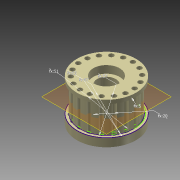
# Autodesk Inventor part: NagyKerek
Saved by Autodesk Inventor 2015 (Build 190159000, 159)
## iProperties
Created: 2014-04-13
Part Number: NagyKerek
Material: Nylon, molybdenum disulphide
Document SubType Name: Modeling
Designer: laca
Density: 1.13 g/cm^3
Appearance: Nylon 6
Mass: 91.8836 g
Surface Area: 251.529 cm^2
Volume: 81.3129 cm^3
Author: laca
Autodesk Inventor part; units mm, degrees
ref_plane "YZ Plane" through (0, 0, 0) normal (1, 0, 0) x (0, 1, 0)
ref_plane "XZ Plane" through (0, 0, 0) normal (0, 1, 0) x (-1, 0, 0)
ref_plane "XY Plane" through (0, 0, 0) normal (0, 0, 1) x (1, 0, 0)
sketch "Sketch1" plane through (0, 0, 0) normal (0, 0, 1) x (1, 0, 0)
  circle A0 centre (0.0338, 1.5) radius 28.5
  arc A1 (-1.1621, 26.972) -> (1.1984, 26.9734) centre (0.0338, 1.5) ccw
  line L0 (-1.1621, 26.972) -> (0.0338, 1.5)
  line L1 (0.0338, 1.5) -> (1.1984, 26.9734)
  arc A2 (1.3007, 29.9718) -> (-1.3028, 29.9687) centre (0.0338, 1.5) ccw
  circle A3 centre (1.3379, 26.9666) radius 2.5
  point P0 (1.3508, 29.9696)
  dimension "d53" = 5
  dimension "d22" = 57
  dimension "d23" = 51
  constraints: 8 point on circle, 4 end point, 3 centre point, 3 coincident, 3 other
  measures "d22" diameter of A0
  measures "d23" diameter of A1
sketch "Sketch2" plane through (0, 0, 0) normal (0, 0, 1) x (1, 0, 0)
  circle A0 centre (0, 0) radius 28.5
  circle A1 centre (0, 0) radius 10
  circle A2 centre (0, 0) radius 31.5
  dimension "d10" = 57
  dimension "d32" = 63
  dimension "d37" = 20
  constraints: 3 centre point, 3 coincident
  measures "d10" diameter of A0
  measures "d32" diameter of A2
  measures "d37" diameter of A1
extrude "Extrusion5" add sketch "Sketch2" along normal blind 31 contours A0
extrude "Extrusion9" add sketch "Sketch2" against normal blind 9 contours A0 | A2
sketch "Sketch3" plane through (0, 0, 31) normal (0, 0, 1) x (1, 0, 0)
  circle A0 centre (0, 0) radius 31.5
  circle A1 centre (0, 0) radius 10
  dimension "d38" = 63
  dimension "d40" = 20
  constraints: 2 centre point, 1 coincident
  measures "d38" diameter of A0
  measures "d40" diameter of A1
extrude "Extrusion11" add sketch "Sketch3" along normal blind 4
extrude "Extrusion15" cut sketch "Sketch1" along normal through all both and the other way through all contours A3 A1 L1 | A3 L1 A1
pattern_circular "Circular Pattern4" count 18 over 360 about axis through (0, 0, 0) along (0, 0, 1) of "Extrusion15"
sketch "Sketch7" plane through (0, 0, -9) normal (0, 0, -1) x (-1, 0, 0)
  circle A0 centre (0, 0) radius 10 projected
  circle A1 centre (0, 0) radius 31.5 projected
  circle A2 centre (0, 0) radius 14
  dimension "d62" = 28
  constraints: 1 centre point, 1 coincident
  measures "d62" diameter of A2
extrude "Extrusion17" cut sketch "Sketch7" against normal blind 27 contours A2
sketch "Sketch8" plane through (0, 0, 35) normal (0, 0, 1) x (1, 0, 0)
  circle A0 centre (0, 0) radius 14
  dimension "d65" = 28
  constraints: 1 centre point, 1 coincident
  measures "d65" diameter of A0
extrude "Extrusion18" cut sketch "Sketch8" against normal blind 8
ref_plane "Work Plane2" through (0, 0, 15.5) normal (0, 0, 1) x (1, 0, 0)
equation "\"d53\" = 2 * SzíjFogakSugaraA"
equation "\"d22\" = 0.5 * NagyKerekAtmero"
equation "\"d23\" = 0.5 * NagyKerekAtmero - 2 * SzíjSugarKözépontEltolásaAzAlaptolA"
equation "\"d10\" = 0.5 * NagyKerekAtmero"
equation "\"d32\" = 0.5 * NagyKerekAtmero + 2 * NagyKerekPeremMagasaga"
equation "\"d37\" = NgyKerekFurat"
equation "\"d15\" = SzíjSzélességB"
equation "\"d38\" = 0.5 * NagyKerekAtmero + 2 * NagyKerekPeremMagasaga"
equation "\"d40\" = NgyKerekFurat"
equation "\"d54\" = NagyKerekPeremSzélesege"
equation "\"d63\" = NagyKerekPeremSzélesege + 0.5 * SzíjSzélességB + 0.5 * KisKerekCSapagySzeleseg"
equation "\"SzíjSzélességA\" = 31"
equation "\"SzíjAlapVastagságA\" = 3"
equation "\"SzíjFogakSugaraA\" = 2.5"
equation "\"SzíjSugarKözépontEltolásaAzAlaptolA\" = 3"
equation "\"NagyKerekAtmero\" = 114"
equation "\"SzíjSzélességB\" = 31"
equation "\"SzíjFogakSugaraB\" = 2.5"
equation "\"SzíjSugarKözépontEltolásaAzAlaptolB\" = 3"
equation "\"SzíjAlapVastagságB\" = 3"
equation "\"NagyKerekPeremSzélesege\" = 4"
equation "\"NagyKerekPeremMagasaga\" = 3"
equation "\"NgyKerekFurat\" = 20"
equation "\"NagyKerekTengelyVastagsag\" = 14"
equation "\"NagyKerékCsapágySzéleseg\" = 15"
equation "\"NagyKerekTengelyVastagság\" = 14"
equation "\"NagyKerékCsapágyBelsőÁtmérő\" = 12"
equation "\"TartoCsőFalVastagsága\" = 2"
equation "\"KisCsoBelsoFalvastagsag\" = 2"
equation "\"OrsoTengelyAtmeroje\" = 8"
equation "\"KisCsaoagyKulsoAtmero\" = 18"
equation "\"CsigaHajtásFogasKerékÁtmérő\" = 56"
equation "\"ZártSzelvényFalVastagság\" = 2"
equation "\"NagyFogaskerekSzelesege\" = 8"
equation "\"LemezVastagsag\" = 2"
equation "\"ZártSzelvényBelsőÁtmérő\" = 12"
equation "\"ForgoTalpKarBeugrasztas\" = 82"
equation "\"KisKerekCSapagySzeleseg\" = 15"
equation "\"NagyKerékSzélesege\" = 75"
body "Solid28"
